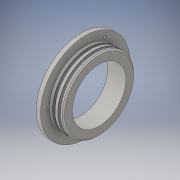
# Autodesk Inventor part: Oring Fitting Dome V3
Saved by Autodesk Inventor 2016 (Build 200138000, 138)
## iProperties
Created: 2017-03-06
Part Number: Oring Fitting Dome V3
Material: Generic
Document SubType Name: Modeling
Designer: Student
Density: 1 g/cm^3
Appearance: Default
Author: Student
Autodesk Inventor part; units mm, degrees
ref_plane "YZ Plane" through (0, 0, 0) normal (1, 0, 0) x (0, 1, 0)
ref_plane "XZ Plane" through (0, 0, 0) normal (0, 1, 0) x (-1, 0, 0)
ref_plane "XY Plane" through (0, 0, 0) normal (0, 0, 1) x (1, 0, 0)
sketch "Sketch1" plane through (0, 0, 0) normal (0, 1, 0) x (-1, 0, 0)
  line L0 (0, 0) -> (4.445, 0)
  line L1 (0, 0) -> (0, -3.175)
  line L2 (0, -3.175) -> (-3.175, -3.175)
  line L3 (-3.175, -3.175) -> (-3.175, 0)
  line L4 (-3.175, 0) -> (-7.62, 0)
  line L5 (-7.62, 0) -> (-7.62, -3.175)
  line L6 (-7.62, -3.175) -> (-10.795, -3.175)
  line L7 (-10.795, -3.175) -> (-10.795, 0)
  line L8 (-10.795, 0) -> (-15.24, 0)
  line L9 (-15.24, 0) -> (-15.24, -12.7)
  line L10 (-15.24, -12.7) -> (4.445, -12.7)
  line L11 (4.445, -12.7) -> (4.445, 0)
  line L12 (-15.24, 0) -> (-15.24, -50.8) construction
  line L13 (-15.24, -50.8) -> (-2.54, -50.8) construction
  dimension "d0" = 4.445
  dimension "d1" = 3.175
  dimension "d2" = 3.175
  dimension "d3" = 4.445
  dimension "d4" = 3.175
  dimension "d5" = 4.445
  dimension "d6" = 12.7
  dimension "d7" = 50.8
  dimension "d36" = 12.7
  dimension "d38" = 12.7
  constraints: 28 end point, 7 perpendicular, 4 point on line, 3 vertical, 2 horizontal
  measures "d0" distance of L0.start L0.end
  measures "d1" distance of L0.start L1.end
  measures "d2" distance of L1.end L2.end
  measures "d3" distance of L3.end L4.end
  measures "d4" distance of L5.end L6.end
  measures "d5" distance of L7.end L8.end
  measures "d6" distance of L8.end L9.end
  measures "d7" distance of L8.end L12.end
  measures "d36" distance of L10.end L0.end
  measures "d38" distance of L12.end L13.end
revolve "Revolution1" add sketch "Sketch1" angle 360 about axis through (15.24, 0, -50.8) along (-1, 0, 0)
sketch "Sketch2" plane through (-4.445, 0, -50.8) normal (-1, 0, 0) x (0, 0, 1)
  circle A0 centre (0, 0) radius 38.1
  circle A1 centre (0, 0) radius 63.5
  circle A2 centre (0, 0) radius 38.1 projected
  dimension "d9" = 76.2
  dimension "d10" = 127
  constraints: 2 centre point, 1 coincident, 1 concentric
  measures "d9" diameter of A0
  measures "d10" diameter of A1
extrude "Extrusion1" add sketch "Sketch2" along normal blind 6.096
sketch "Sketch3" plane through (-10.541, 0, -50.8) normal (-1, 0, 0) x (0, 0, 1)
  circle A0 centre (0, 0) radius 49.0093
  circle A1 centre (0, 0) radius 52.1843
  circle A2 centre (0, 0) radius 38.1 projected
  dimension "d41" = 10.9093
  dimension "d42" = 3.175
  constraints: 2 centre point, 2 coincident
  measures "d41" radial gap between concentric circles of A2 A0
  measures "d42" radial gap between concentric circles of A1 A0
extrude "Extrusion2" cut sketch "Sketch3" against normal blind 3.5306 contours A1
chamfer "Chamfer1" distance 1.778 angle 45 1 edges at (15.24, 0, -101.6)
sketch "Sketch5" plane through (-10.541, 0, -50.8) normal (-1, 0, 0) x (0, 0, 1)
  circle A0 centre (0, 0) radius 55.245 construction
  circle A1 centre (0, 0) radius 38.1 projected
  point P0 (-55.245, 0)
  point P1 (-27.6225, -47.8436)
  point P2 (27.6225, -47.8436)
  point P3 (55.245, 0)
  point P4 (27.6225, 47.8436)
  point P5 (-27.6225, 47.8436)
  dimension "d43" = 110.49
  dimension "d46" = 360
  constraints: 1 horizontal alignment, 10 other
hole "Hole1" at (-10.541, 0, -106.045) at (-10.541, -47.8436, -78.4225) at (-10.541, -47.8436, -23.1775) at (-10.541, 0, 4.445) at (-10.541, 47.8436, -23.1775) at (-10.541, 47.8436, -78.4225) direction (1, 0, 0) diameter 3.5052 end through all
chamfer "Chamfer2" distance 0.254 angle 45 6 edges at (0, 0, -101.6) (3.175, 0, -101.6) (7.62, 0, -101.6) (10.795, 0, -101.6) (-10.541, 0, -102.9843) (-10.541, 0, -99.8093)
body "Solid1"
